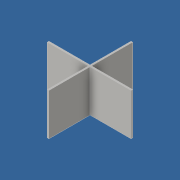
# Autodesk Inventor part: Case Button Jig
Saved by Autodesk Inventor 2016 (Build 200138000, 138)
## iProperties
Created: 2016-01-04
Part Number: Case Button Jig
Material: Generic
Document SubType Name: Modeling
Designer: Sam Clay
Density: 1 g/cm^3
Appearance: Default
Author: Sam Clay
Autodesk Inventor part; units mm, degrees
ref_plane "YZ Plane" through (0, 0, 0) normal (1, 0, 0) x (0, 1, 0)
ref_plane "XZ Plane" through (0, 0, 0) normal (0, 1, 0) x (-1, 0, 0)
ref_plane "XY Plane" through (0, 0, 0) normal (0, 0, 1) x (1, 0, 0)
sketch "Sketch1" plane through (0, 0, 0) normal (0, 1, 0) x (-1, 0, 0)
  line L0 (-0.254, 12.7) -> (-0.254, -12.7)
  line L1 (-0.254, -12.7) -> (0.254, -12.7)
  line L2 (0.254, -12.7) -> (0.254, 12.7)
  line L3 (0.254, 12.7) -> (-0.254, 12.7)
  line L4 (-0.254, 12.7) -> (0.254, -12.7) construction
  line L5 (-0.254, -12.7) -> (0.254, 12.7) construction
  line L6 (12.7, 0.254) -> (-12.7, 0.254)
  line L7 (-12.7, 0.254) -> (-12.7, -0.254)
  line L8 (-12.7, -0.254) -> (12.7, -0.254)
  line L9 (12.7, -0.254) -> (12.7, 0.254)
  line L10 (12.7, 0.254) -> (-12.7, -0.254) construction
  line L11 (-12.7, 0.254) -> (12.7, -0.254) construction
  point P0 (0, 0)
  dimension "d0" = 25.4
  dimension "d1" = 0.508
  dimension "d2" = 25.4
  dimension "d3" = 0.508
  constraints: 24 end point, 5 parallel, 4 midpoint, 2 perpendicular, 1 vertical
  measures "d0" distance of L0.start L0.end
  measures "d1" distance of L1.end L0.end
  measures "d2" distance of L6.start L6.end
  measures "d3" distance of L7.end L6.end
extrude "Extrusion1" add sketch "Sketch1" along normal blind 12.7
body "Solid1"
